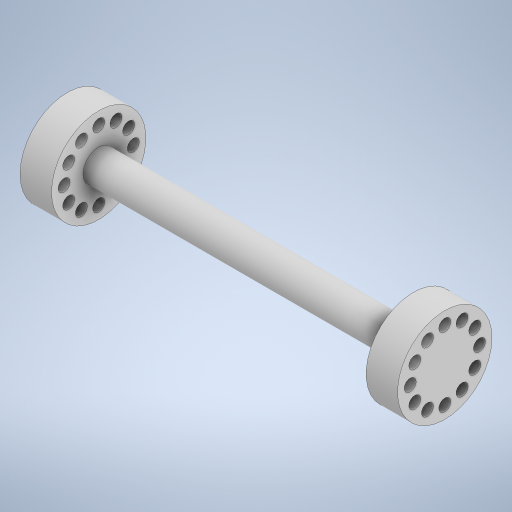
# Autodesk Inventor part: ferris_wheel_central_hub
Saved by Autodesk Inventor 2023 (Build 270158000, 158)
## iProperties
Created: 2025-10-18
Part Number: ferris_wheel_central_hub
Material: Generic
Document SubType Name: Modeling
Designer: Justin Pascual
Density: 1 g/cm^3
Appearance: Default
Author: Justin Pascual
Autodesk Inventor part; units mm, degrees
ref_plane "YZ Plane" through (0, 0, 0) normal (1, 0, 0) x (0, 1, 0)
ref_plane "XZ Plane" through (0, 0, 0) normal (0, 1, 0) x (-1, 0, 0)
ref_plane "XY Plane" through (0, 0, 0) normal (0, 0, 1) x (1, 0, 0)
sketch "Sketch1" plane through (0, 0, 0) normal (1, 0, 0) x (0, 1, 0)
  circle A0 centre (0, 0) radius 3.175
  dimension "d0" = 6.35
  constraints: 1 centre point, 1 coincident
  measures "d0" diameter of A0
extrude "Extrusion1" add sketch "Sketch1" along normal blind 63.5
sketch "Sketch2" plane through (63.5, 0, 0) normal (1, 0, 0) x (0, 0, -1)
  circle A0 centre (0, 0) radius 9.525
  dimension "d3" = 19.05
  constraints: 1 centre point, 1 coincident
  measures "d3" diameter of A0
extrude "Extrusion2" add sketch "Sketch2" along normal blind 6.35
sketch "Sketch3" plane through (0, 0, 0) normal (-1, 0, 0) x (0, 0, 1)
  circle A0 centre (0, 0) radius 9.525
  dimension "d6" = 19.05
  constraints: 1 centre point, 1 coincident
  measures "d6" diameter of A0
extrude "Extrusion3" add sketch "Sketch3" along normal blind 6.35
sketch "Sketch4" plane through (-6.35, 0, 0) normal (-1, 0, 0) x (0, 0, 1)
  point P0 (0, 0)
  point P1 (0, -6.985)
  dimension "d9" = 6.985
  measures "d9" distance of point (0, -6.985) point (0, 0)
hole "Hole1" at (-6.35, -6.985, 0) direction (1, 0, 0) diameter 2.4384 end through all clearance for "Flat Head Machine Screw (82)" size "#2" standard "Ansi Unified Screw Threads"
pattern_circular "Circular Pattern1" count 12 over 360 about axis through (0, 0, 0) along (-1, 0, 0) of "Hole1"
body "Solid1"
